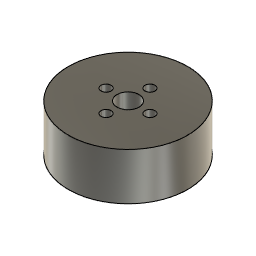
disc (Autodesk Fusion 360 design; units mm, degrees)
Autodesk Fusion 360 part; units mm, degrees
sketch "Sketch1" plane through (0, 0, 0) normal (0, 0, 1) x (1, 0, 0)
  circle A0 centre (0, 0) radius 19
  line L0 (0, 30.1169) -> (0, -30.2243) construction
  line L1 (0, 0) -> (0, 7.5) construction
  circle A1 centre (0, 7.5) radius 0.8 construction
  line L2 (0, 0) -> (0, 10.5) construction
  circle A2 centre (0, 10.5) radius 0.8 construction
  line L3 (0, 0) -> (0, 13.5) construction
  circle A3 centre (0, 13.5) radius 0.8 construction
  line L4 (0, 0) -> (0, 16.5) construction
  circle A4 centre (0, 16.5) radius 0.8 construction
  circle A5 centre (-6.4952, 3.75) radius 0.8 construction
  circle A6 centre (-9.0933, 5.25) radius 0.8 construction
  circle A7 centre (-11.6913, 6.75) radius 0.8 construction
  circle A8 centre (-14.2894, 8.25) radius 0.8 construction
  circle A9 centre (-6.4952, -3.75) radius 0.8 construction
  circle A10 centre (-9.0933, -5.25) radius 0.8 construction
  circle A11 centre (-11.6913, -6.75) radius 0.8 construction
  circle A12 centre (-14.2894, -8.25) radius 0.8 construction
  circle A13 centre (0, -7.5) radius 0.8 construction
  circle A14 centre (0, -10.5) radius 0.8 construction
  circle A15 centre (0, -13.5) radius 0.8 construction
  circle A16 centre (0, -16.5) radius 0.8 construction
  circle A17 centre (6.4952, -3.75) radius 0.8 construction
  circle A18 centre (9.0933, -5.25) radius 0.8 construction
  circle A19 centre (11.6913, -6.75) radius 0.8 construction
  circle A20 centre (14.2894, -8.25) radius 0.8 construction
  circle A21 centre (6.4952, 3.75) radius 0.8 construction
  circle A22 centre (9.0933, 5.25) radius 0.8 construction
  circle A23 centre (11.6913, 6.75) radius 0.8 construction
  circle A24 centre (14.2894, 8.25) radius 0.8 construction
  circle A25 centre (-7.5, 0) radius 0.8 construction
  circle A26 centre (-10.5, 0) radius 0.8 construction
  circle A27 centre (-13.5, 0) radius 0.8 construction
  circle A28 centre (-16.5, 0) radius 0.8 construction
  circle A29 centre (7.5, 0) radius 0.8 construction
  circle A30 centre (10.5, 0) radius 0.8 construction
  circle A31 centre (13.5, 0) radius 0.8 construction
  circle A32 centre (16.5, 0) radius 0.8 construction
  line L5 (0, 0) -> (7, 0) construction
  circle A33 centre (7, 0) radius 1.6
  circle A34 centre (0, 7) radius 1.6
  circle A35 centre (-7, 0) radius 1.6
  circle A36 centre (0, -7) radius 1.6
  circle A37 centre (0, 0) radius 3.5
  dimension "d1" = 38
  dimension "d16" = 7.5
  dimension "d17" = 1.6
  dimension "d18" = 10.5
  dimension "d19" = 1.6
  dimension "d20" = 13.5
  dimension "d21" = 1.6
  dimension "d22" = 16.5
  dimension "d23" = 1.6
  dimension "d25" = 360
  dimension "d27" = 90
  dimension "d28" = 7
  dimension "d29" = 3.2
  dimension "d31" = 360
  dimension "d32" = 7
  constraint coincident A0.centre L1.start
  constraint vertical L0
  constraint coincident L0 L1.end
  constraint parallel L0 L1
  constraint coincident L1.end A1.centre
  constraint coincident L0 L2.end
  constraint coincident L2.end A2.centre
  constraint coincident L0 L3.end
  constraint coincident L3.end A3.centre
  constraint coincident L0 L4.end
  constraint coincident L4.end A4.centre
  constraint symmetric L0 A25 A29
  constraint symmetric L0 A26 A30
  constraint symmetric L0 A27 A31
  constraint symmetric L0 A28 A32
  constraint perpendicular L2 L5
  constraint coincident L5.end A33.centre
  constraint concentric A0 A37
  measures "d1" diameter of A0
  measures "d16" distance of A0.centre L1.end
  measures "d17" diameter of A1
  measures "d18" distance of A0.centre L2.end
  measures "d19" diameter of A2
  measures "d20" distance of A0.centre L3.end
  measures "d21" diameter of A3
  measures "d22" distance of A0.centre L4.end
  measures "d23" diameter of A4
  measures "d28" distance of A0.centre L5.end
  measures "d29" diameter of A33
  measures "d32" diameter of A37
extrude "Extrude1" add sketch "Sketch1" along normal blind 15
equation "d16 = ( 15 / 2 ) * 1 mm"
equation "d18 = ( 21 / 2 ) * 1 mm"
equation "d20 = ( 27 / 2 ) * 1 mm"
equation "d22 = ( 33 / 2 ) * 1 mm"
equation "d28 = ( 14 / 2 ) * 1 mm"
